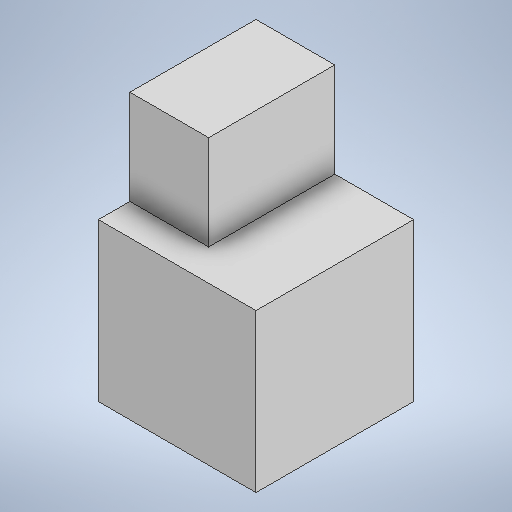
# Autodesk Inventor part: two_blocks
Saved by Autodesk Inventor 2025 (Build 290162000, 162)
## iProperties
Created: 2024-09-07
Part Number: two_blocks
Material: Generic
Document SubType Name: Modeling
Designer: au621298
Density: 1 g/cm^3
Appearance: Default
Author: au621298
Autodesk Inventor part; units mm, degrees
ref_plane "YZ Plane" through (0, 0, 0) normal (1, 0, 0) x (0, 1, 0)
ref_plane "XZ Plane" through (0, 0, 0) normal (0, 1, 0) x (-1, 0, 0)
ref_plane "XY Plane" through (0, 0, 0) normal (0, 0, 1) x (1, 0, 0)
sketch "Sketch1" plane through (0, 0, 0) normal (0, 1, 0) x (-1, 0, 0)
  line L0 (0, 0) -> (10, 0)
  line L1 (10, 0) -> (10, -10)
  line L2 (10, -10) -> (0, -10)
  line L3 (0, -10) -> (0, 0)
  dimension "d0" = 10
  dimension "d1" = 10
  constraints: 8 end point, 2 parallel, 1 horizontal, 1 perpendicular
  measures "d0" distance of L0.end L1.end
  measures "d1" distance of L1.end L2.end
extrude "Extrusion1" add sketch "Sketch1" along normal blind 10
sketch "Sketch2" plane through (0, 10, 0) normal (0, 1, 0) x (1, 0, 0)
  line L0 (0, 10) -> (-10, 10) projected
  line L1 (-10, 10) -> (-10, 0) projected
  line L2 (-10, 0) -> (0, 0) projected
  line L3 (0, 0) -> (0, 10) projected
  line L4 (-10, 10) -> (-5, 10)
  line L5 (-5, 10) -> (-5, 2)
  line L6 (-5, 2) -> (-10, 2)
  line L7 (-10, 2) -> (-10, 10)
  dimension "d4" = 5
  dimension "d5" = 8
  constraints: 8 end point, 2 parallel, 1 horizontal, 1 perpendicular
  measures "d4" distance of L5.end L6.end
  measures "d5" distance of L4.end L5.end
extrude "Extrusion2" cut sketch "Sketch2" against normal blind 4 contours L5 L6 L1 L0
sketch "Sketch3" plane through (0, 6, 0) normal (0, 1, 0) x (1, 0, 0)
  line L0 (-5, 10) -> (-5, 2) projected
  line L1 (-10, 10) -> (-5, 10) projected
  line L2 (-10, 2) -> (-10, 10) projected
  line L3 (-5, 2) -> (-10, 2) projected
  point P0 (0, 0)
extrude "Extrusion3" add sketch "Sketch3" along normal blind 10 separate body
equation "\"d1\" = d0"
body "Solid1"
body "Solid2"
